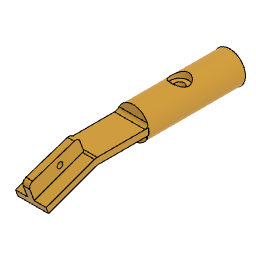
Figure-6 (Autodesk Fusion 360 design; units mm, degrees)
Autodesk Fusion 360 part; units mm, degrees
sketch "Sketch1" plane through (0, 0, 0) normal (0, 1, 0) x (1, 0, 0)
  circle A0 centre (0, 0) radius 14
  dimension "d1" = 28
  constraint coincident A0.centre origin
  measures "d1" diameter of A0
extrude "Extrude1" add sketch "Sketch1" along normal blind 86
sketch "Sketch2" plane through (0, 0, 0) normal (0, 1, 0) x (1, 0, 0)
  point P0 (-14, 0)
sketch "Sketch4" plane through (0, 0, 0) normal (0, 0, 1) x (1, 0, 0)
  point P0 (-14, 0)
hole "Hole1" at (0, 41.3975, 14) direction (0, 0, -1) diameter 8 depth 28 tip angle 180 counterbore diameter 16 counterbore depth 6
sketch "Sketch6" plane through (0, 0, 0) normal (1, 0, 0) x (0, 1, 0)
  line L0 (0, 3) -> (-1, 3)
  line L1 (-1, 3) -> (-47, 3)
  line L2 (-47, 3) -> (-91.1673, -13.0701)
  line L3 (-91.1673, -13.0701) -> (-89.1158, -18.7085)
  line L4 (-89.1158, -18.7085) -> (-45.9424, -3)
  line L5 (0, 3) -> (0, -3)
  line L6 (0, -3) -> (-45.9424, -3)
  line L7 (-91.1673, -13.0701) -> (-91.643, -11.7627)
  line L8 (-91.643, -11.7627) -> (-96.4299, 1.3935)
  line L9 (-47, 3) -> (-51.7868, 16.1562)
  line L10 (-51.7868, 16.1562) -> (-96.4299, 1.3935)
  circle A0 centre (-68.188, 2.7398) radius 2.5
  dimension "d23" = 46
  dimension "d24" = 47
  dimension "d25" = 6
  dimension "d27" = 6
  dimension "d28" = 14
  dimension "d29" = 14
  dimension "d33" = 5
  dimension "d34" = 20
  dimension "d35" = 7
  constraint horizontal L0
  constraint parallel L0 L1
  constraint perpendicular L2 L3
  constraint perpendicular L3 L4
  constraint perpendicular L0 L5
  constraint perpendicular L5 L6
  constraint coincident origin L5
  constraint midpoint origin L5
  constraint perpendicular L2 L7
  constraint perpendicular L2 L8
  constraint perpendicular L2 L9
  measures "d23" distance of L0.end L1.end
  measures "d24" distance of L1.end L2.end
  measures "d25" distance of L2.end L3.end
  measures "d27" distance of L0.start L5.end
  measures "d28" distance of L7.end L8.end
  measures "d29" distance of L1.end L9.end
  measures "d33" diameter of A0
  measures "d34" distance of L9 A0.centre
  measures "d35" distance of L2 A0.centre
extrude "Extrude2" add sketch "Sketch6" along normal mid plane 27.35 contours L0 L1 L2 L3 L4 L5 L6
fillet "Fillet1" radius 3 2 edges at (0, 0, 3) (0, 0, -3)
fillet "Fillet2" radius 7 2 edges at (0, -47, 3) (0, -45.9424, -3)
extrude "Extrude3" add sketch "Sketch6" along normal mid plane 6 contours L2 L7 L8 L9 L10
fillet "Fillet3" radius 4 2 edges at (0, -51.7868, 16.1562) (0, -96.4299, 1.3935)
